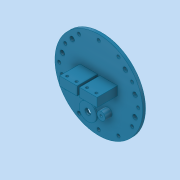
# Autodesk Inventor part: frontServoAttachmentPlate
Saved by Autodesk Inventor 2017 (Build 210142000, 142)
## iProperties
Created: 2016-10-29
Part Number: frontServoAttachmentPlate
Material: ABS Plastic
Document SubType Name: Modeling
Designer: techn
Density: 1.06 g/cm^3
Appearance: Sky Blue Dark
Mass: 31.7141 g
Surface Area: 183.858 cm^2
Volume: 29.9189 cm^3
Author: techn
Autodesk Inventor part; units mm, degrees
ref_plane "YZ Plane" through (0, 0, 0) normal (1, 0, 0) x (0, 1, 0)
ref_plane "XZ Plane" through (0, 0, 0) normal (0, 1, 0) x (-1, 0, 0)
ref_plane "XY Plane" through (0, 0, 0) normal (0, 0, 1) x (1, 0, 0)
sketch "Sketch1" plane through (0, 0, 0) normal (0, 0, 1) x (1, 0, 0)
  circle A0 centre (0, 0) radius 47.625
  dimension "d0" = 95.25
  constraints: 1 centre point, 1 coincident
  measures "d0" diameter of A0
extrude "Extrusion1" add sketch "Sketch1" along normal blind 3.175
sketch "Sketch3" plane through (0, 0, 3.175) normal (0, 0, 1) x (1, 0, 0)
  line L0 (1.27, 9.525) -> (20.32, 9.525)
  line L1 (20.32, 9.525) -> (20.32, 0)
  line L2 (20.32, 0) -> (1.27, 0)
  line L3 (1.27, 0) -> (1.27, 9.525)
  line L4 (0, 0) -> (0, -11.0035)
  line L5 (-1.27, 9.525) -> (-20.32, 9.525)
  line L6 (-20.32, 9.525) -> (-20.32, 0)
  line L7 (-20.32, 0) -> (-1.27, 0)
  line L8 (-1.27, 0) -> (-1.27, 9.525)
  dimension "d11" = 19.05
  dimension "d12" = 9.525
  dimension "d13" = 1.27
  dimension "d14" = 0
  constraints: 18 end point, 4 symmetric about line, 2 parallel, 1 horizontal, 1 perpendicular, 1 vertical
  measures "d11" distance of L1.end L2.end
  measures "d12" distance of L0.end L1.end
  measures "d13" distance from line of L3 L4.start
  measures "d14" distance from line of L2 L4.start
extrude "Extrusion3" add sketch "Sketch3" along normal blind 22.225
sketch "Sketch4" plane through (1.27, 9.525, 3.175) normal (0, 1, 0) x (1, 0, 0)
  circle A0 centre (4.445, -18.415) radius 1.397
  line L0 (19.05, -22.225) -> (0, -22.225) projected
  circle A1 centre (14.605, -18.415) radius 1.397
  line L1 (9.525, -22.225) -> (9.525, -7.9119)
  line L2 (-1.27, 3.175) -> (-1.27, 8.3959)
  circle A2 centre (-6.985, -18.415) radius 1.397
  circle A3 centre (-17.145, -18.415) radius 1.397
  dimension "d17" = 2.794
  dimension "d18" = 3.81
  dimension "d19" = 2.794
  dimension "d20" = 3.81
  dimension "d21" = 10.16
  dimension "d22" = 5.08
  constraints: 4 centre point, 4 end point, 2 symmetric about line, 2 vertical, 1 midpoint, 2 other
  measures "d17" diameter of A0
  measures "d18" distance from line of L0 A0.centre
  measures "d19" diameter of A1
  measures "d20" distance from line of L0 A1.centre
  measures "d21" distance of A1.centre A0.centre
  measures "d22" distance from line of L1 A0.centre
extrude "Extrusion4" cut sketch "Sketch4" against normal through all
sketch "Sketch5" plane through (0, 0, 0) normal (0, 0, -1) x (-1, 0, 0)
  circle A0 centre (10.541, -29.7561) radius 3.25
  point P0 (0, 0)
  dimension "d25" = 6.5
  dimension "d26" = 10.541
  dimension "d27" = 29.7561
  constraints: 1 centre point
  measures "d25" diameter of A0
  measures "d26" horizontal distance of point (0, 0) A0.centre
  measures "d27" vertical distance of point (0, 0) A0.centre
extrude "Extrusion5" cut sketch "Sketch5" against normal blind 25.4
sketch "Sketch6" plane through (0, 0, 3.175) normal (0, 0, 1) x (1, 0, 0)
  circle A0 centre (-10.541, -29.7561) radius 3.25 projected
  circle A1 centre (0, 0) radius 47.625 projected
  circle A2 centre (-10.541, -29.7561) radius 9.525
  dimension "d30" = 19.05
  constraints: 1 centre point, 1 coincident
  measures "d30" diameter of A2
extrude "Extrusion6" add sketch "Sketch6" along normal blind 1.27 contours A2
sketch "Sketch7" plane through (0, 0, 0) normal (0, 0, -1) x (-1, 0, 0)
  circle A0 centre (10.541, -29.7561) radius 3.25 projected
  circle A1 centre (0, 0) radius 47.625 projected
  line L0 (5.0564, -29.7561) -> (7.7987, -25.0063)
  line L1 (7.7987, -25.0063) -> (13.2833, -25.0063)
  line L2 (13.2833, -25.0063) -> (16.0256, -29.7561)
  line L3 (16.0256, -29.7561) -> (13.2833, -34.5059)
  line L4 (13.2833, -34.5059) -> (7.7987, -34.5059)
  line L5 (7.7987, -34.5059) -> (5.0564, -29.7561)
  dimension "d33" = 9.4996
  constraints: 12 end point, 1 coincident, 13 other
  measures "d33" distance between parallel lines of L4 L1
extrude "Extrusion7" cut sketch "Sketch7" against normal blind 2.54 contours L0 L1 L2 L3 L4 L5
sketch "Sketch9" plane through (0, 0, 0) normal (0, 0, -1) x (-1, 0, 0)
  line L0 (0, 0) -> (21.4313, 37.12)
  line L1 (0, 0) -> (42.8625, 0) construction
  circle A0 centre (21.4313, 37.12) radius 1.8415
  circle A1 centre (-21.4312, 37.12) radius 1.8415
  circle A2 centre (-42.8625, 0) radius 1.8415
  circle A3 centre (-21.4313, -37.12) radius 1.8415
  circle A4 centre (21.4312, -37.12) radius 1.8415
  circle A5 centre (42.8625, 0) radius 1.8415
  dimension "d44" = 42.8625
  dimension "d45" = 60
  dimension "d46" = 3.683
  dimension "d49" = 360
  constraints: 6 centre point, 4 end point, 1 coincident, 1 equal length, 1 horizontal, 13 other
  measures "d44" distance of L0.start L0.end
  measures "d45" angle of L1 L0
  measures "d46" diameter of A0
extrude "Extrusion9" cut sketch "Sketch9" against normal blind 25.4
sketch "Sketch10" plane through (0, 0, 3.175) normal (0, 0, 1) x (1, 0, 0)
  line L0 (0, 0) -> (0, 41.91)
  circle A0 centre (0, 41.91) radius 1.8415
  circle A1 centre (-36.2951, 20.955) radius 1.8415
  circle A2 centre (-36.2951, -20.955) radius 1.8415
  circle A3 centre (0, -41.91) radius 1.8415
  circle A4 centre (36.2951, -20.955) radius 1.8415
  circle A5 centre (36.2951, 20.955) radius 1.8415
  dimension "d53" = 41.91
  dimension "d54" = 3.683
  dimension "d57" = 360
  constraints: 6 centre point, 2 end point, 1 coincident, 1 vertical, 13 other
  measures "d53" distance of L0.start L0.end
  measures "d54" diameter of A0
extrude "Extrusion10" cut sketch "Sketch10" against normal blind 25.4
sketch "Sketch11" plane through (0, 0, 3.175) normal (0, 0, 1) x (1, 0, 0)
  line L0 (0, 0) -> (39.3779, 10.5513)
  line L1 (0, 0) -> (40.767, 0) construction
  circle A0 centre (39.3779, 10.5513) radius 2.54
  line L2 (0, 0) -> (0, 16.7096)
  circle A1 centre (39.3779, -10.5513) radius 2.54
  line L3 (0, 0) -> (-40.767, 0) construction
  circle A2 centre (-39.3779, 10.5513) radius 2.54
  circle A3 centre (-39.3779, -10.5513) radius 2.54
  line L4 (0, 0) -> (28.8266, 28.8266)
  line L5 (0, 0) -> (40.767, 0) construction
  circle A4 centre (28.8266, 28.8266) radius 2.54
  circle A5 centre (-28.8266, 28.8266) radius 2.54
  dimension "d61" = 40.767
  dimension "d62" = 15
  dimension "d63" = 5.08
  dimension "d66" = 40.767
  dimension "d67" = 45
  dimension "d68" = 5.08
  constraints: 12 end point, 6 centre point, 5 symmetric about line, 2 coincident, 2 equal length, 2 horizontal, 1 vertical, 4 other
  measures "d61" distance of L0.start L0.end
  measures "d62" angle of L1 L0
  measures "d63" diameter of A0
  measures "d66" distance of L0.start L4.end
  measures "d67" angle of L5 L4
  measures "d68" diameter of A4
extrude "Extrusion11" cut sketch "Sketch11" against normal blind 25.4 contours A0 | A1 | A2 | A3
extrude "Extrusion12" cut sketch "Sketch11" against normal blind 25.4 contours A4 | A5
sketch "Sketch12" plane through (0, 0, 3.175) normal (0, 0, 1) x (1, 0, 0)
  circle A0 centre (10.16, -20.32) radius 1.397
  circle A1 centre (10.16, -20.32) radius 4.445
  point P0 (0, 0)
  dimension "d71" = 2.794
  dimension "d72" = 8.89
  dimension "d73" = 20.32
  dimension "d74" = 10.16
  constraints: 2 centre point, 1 coincident
  measures "d71" diameter of A0
  measures "d72" diameter of A1
  measures "d73" vertical distance of A0.centre point (0, 0)
  measures "d74" horizontal distance of A0.centre point (0, 0)
extrude "Extrusion13" add sketch "Sketch12" along normal blind 7.62
body "Solid1"
